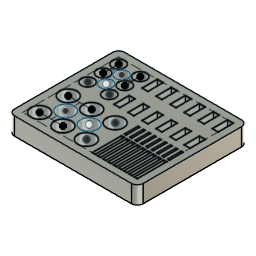
microSD-SD-flashdrive-AA-AAA holder final version. v1 (Autodesk Fusion 360 design; units mm, degrees)
Autodesk Fusion 360 part; units mm, degrees
sketch "Sketch1" plane through (0, 0, 0) normal (0, 0, 1) x (1, 0, 0)
  line L0 (55, 47) -> (-55, 47)
  line L1 (-55, 47) -> (-55, -47)
  line L2 (-55, -47) -> (55, -47)
  line L3 (55, -47) -> (55, 47)
  line L4 (55, 47) -> (-55, -47) construction
  line L5 (-55, 47) -> (55, -47) construction
  dimension "d1" = 110
  dimension "d2" = 94
  constraint horizontal L0
  constraint perpendicular L0 L1
  constraint parallel L0 L2
  constraint parallel L1 L3
  constraint coincident L4 origin
  constraint coincident L5 origin
  measures "d1" distance of L0.start L0.end
  measures "d2" distance of L0.end L1.end
extrude "Extrude1" add sketch "Sketch1" along normal blind 15
sketch "Sketch2" plane through (0, 0, 15) normal (0, 0, 1) x (-1, 0, 0)
  line L0 (-55, 47) -> (-55, -47)
  line L1 (-55, -47) -> (55, -47)
  line L2 (55, -47) -> (55, 47)
  line L3 (55, 47) -> (-55, 47)
  line L4 (49, -41) -> (-49, -41) construction
  line L5 (-49, -41) -> (-49, 41) construction
  line L6 (-49, 41) -> (49, 41) construction
  line L7 (49, 41) -> (49, -41) construction
  line L8 (-49, -41) -> (-44, -41)
  line L9 (-44, -41) -> (-44, -28)
  line L10 (-44, -28) -> (-49, -28)
  line L11 (-49, -28) -> (-49, -41)
  line L12 (-32, -41) -> (-32, -28)
  line L13 (-32, -28) -> (-37, -28)
  line L14 (-37, -28) -> (-37, -41)
  line L15 (-37, -41) -> (-32, -41)
  line L16 (-20, -41) -> (-20, -28)
  line L17 (-20, -28) -> (-25, -28)
  line L18 (-25, -28) -> (-25, -41)
  line L19 (-25, -41) -> (-20, -41)
  line L20 (-8, -41) -> (-8, -28)
  line L21 (-8, -28) -> (-13, -28)
  line L22 (-13, -28) -> (-13, -41)
  line L23 (-13, -41) -> (-8, -41)
  line L24 (4, -41) -> (4, -28)
  line L25 (4, -28) -> (-1, -28)
  line L26 (-1, -28) -> (-1, -41)
  line L27 (-1, -41) -> (4, -41)
  line L28 (16, -41) -> (16, -28)
  line L29 (16, -28) -> (11, -28)
  line L30 (11, -28) -> (11, -41)
  line L31 (11, -41) -> (16, -41)
  line L32 (-44, -17) -> (-44, -4)
  line L33 (-44, -4) -> (-49, -4)
  line L34 (-49, -4) -> (-49, -17)
  line L35 (-49, -17) -> (-44, -17)
  line L36 (-32, -17) -> (-32, -4)
  line L37 (-32, -4) -> (-37, -4)
  line L38 (-37, -4) -> (-37, -17)
  line L39 (-37, -17) -> (-32, -17)
  line L40 (-20, -17) -> (-20, -4)
  line L41 (-20, -4) -> (-25, -4)
  line L42 (-25, -4) -> (-25, -17)
  line L43 (-25, -17) -> (-20, -17)
  line L44 (-8, -17) -> (-8, -4)
  line L45 (-8, -4) -> (-13, -4)
  line L46 (-13, -4) -> (-13, -17)
  line L47 (-13, -17) -> (-8, -17)
  line L48 (4, -17) -> (4, -4)
  line L49 (4, -4) -> (-1, -4)
  line L50 (-1, -4) -> (-1, -17)
  line L51 (-1, -17) -> (4, -17)
  line L52 (16, -17) -> (16, -4)
  line L53 (16, -4) -> (11, -4)
  line L54 (11, -4) -> (11, -17)
  line L55 (11, -17) -> (16, -17)
  line L56 (-49, 2) -> (-47.5, 2)
  line L57 (-47.5, 2) -> (-47.5, 13.5)
  line L58 (-47.5, 13.5) -> (-49, 13.5)
  line L59 (-49, 13.5) -> (-49, 2)
  line L60 (-44.375, 2) -> (-42.875, 2)
  line L61 (-42.875, 2) -> (-42.875, 13.5)
  line L62 (-42.875, 13.5) -> (-44.375, 13.5)
  line L63 (-44.375, 13.5) -> (-44.375, 2)
  line L64 (-39.75, 2) -> (-38.25, 2)
  line L65 (-38.25, 2) -> (-38.25, 13.5)
  line L66 (-38.25, 13.5) -> (-39.75, 13.5)
  line L67 (-39.75, 13.5) -> (-39.75, 2)
  line L68 (-35.125, 2) -> (-33.625, 2)
  line L69 (-33.625, 2) -> (-33.625, 13.5)
  line L70 (-33.625, 13.5) -> (-35.125, 13.5)
  line L71 (-35.125, 13.5) -> (-35.125, 2)
  line L72 (-30.5, 2) -> (-29, 2)
  line L73 (-29, 2) -> (-29, 13.5)
  line L74 (-29, 13.5) -> (-30.5, 13.5)
  line L75 (-30.5, 13.5) -> (-30.5, 2)
  line L76 (-25.875, 2) -> (-24.375, 2)
  line L77 (-24.375, 2) -> (-24.375, 13.5)
  line L78 (-24.375, 13.5) -> (-25.875, 13.5)
  line L79 (-25.875, 13.5) -> (-25.875, 2)
  line L80 (-21.25, 2) -> (-19.75, 2)
  line L81 (-19.75, 2) -> (-19.75, 13.5)
  line L82 (-19.75, 13.5) -> (-21.25, 13.5)
  line L83 (-21.25, 13.5) -> (-21.25, 2)
  line L84 (-16.625, 2) -> (-15.125, 2)
  line L85 (-15.125, 2) -> (-15.125, 13.5)
  line L86 (-15.125, 13.5) -> (-16.625, 13.5)
  line L87 (-16.625, 13.5) -> (-16.625, 2)
  line L88 (-12, 2) -> (-10.5, 2)
  line L89 (-10.5, 2) -> (-10.5, 13.5)
  line L90 (-10.5, 13.5) -> (-12, 13.5)
  line L91 (-12, 13.5) -> (-12, 2)
  line L92 (-49, 16) -> (-46.5, 16)
  line L93 (-46.5, 16) -> (-46.5, 41)
  line L94 (-46.5, 41) -> (-49, 41)
  line L95 (-49, 41) -> (-49, 16)
  line L96 (-42, 16) -> (-42, 41)
  line L97 (-44.5, 16) -> (-42, 16)
  line L98 (-42, 41) -> (-44.5, 41)
  line L99 (-44.5, 41) -> (-44.5, 16)
  line L100 (-37.5, 16) -> (-37.5, 41)
  line L101 (-40, 16) -> (-37.5, 16)
  line L102 (-37.5, 41) -> (-40, 41)
  line L103 (-40, 41) -> (-40, 16)
  line L104 (-33, 16) -> (-33, 41)
  line L105 (-35.5, 16) -> (-33, 16)
  line L106 (-33, 41) -> (-35.5, 41)
  line L107 (-35.5, 41) -> (-35.5, 16)
  line L108 (-28.5, 16) -> (-28.5, 41)
  line L109 (-31, 16) -> (-28.5, 16)
  line L110 (-28.5, 41) -> (-31, 41)
  line L111 (-31, 41) -> (-31, 16)
  line L112 (-24, 16) -> (-24, 41)
  line L113 (-26.5, 16) -> (-24, 16)
  line L114 (-24, 41) -> (-26.5, 41)
  line L115 (-26.5, 41) -> (-26.5, 16)
  line L116 (-19.5, 16) -> (-19.5, 41)
  line L117 (-22, 16) -> (-19.5, 16)
  line L118 (-19.5, 41) -> (-22, 41)
  line L119 (-22, 41) -> (-22, 16)
  line L120 (-15, 16) -> (-15, 41)
  line L121 (-17.5, 16) -> (-15, 16)
  line L122 (-15, 41) -> (-17.5, 41)
  line L123 (-17.5, 41) -> (-17.5, 16)
  line L124 (-10.5, 16) -> (-10.5, 41)
  line L125 (-13, 16) -> (-10.5, 16)
  line L126 (-10.5, 41) -> (-13, 41)
  line L127 (-13, 41) -> (-13, 16)
  circle A0 centre (43.75, -35.75) radius 5.25
  circle A1 centre (25.25, -35.75) radius 5.25
  circle A2 centre (43.75, -22.5) radius 5.25
  circle A3 centre (25.25, -22.5) radius 5.25
  circle A4 centre (43.75, -9.25) radius 5.25
  circle A5 centre (25.25, -9.25) radius 5.25
  line L128 (43.75, -35.75) -> (43.75, -22.5)
  line L129 (25.25, -35.75) -> (25.25, -22.5)
  circle A6 centre (34.5, -29.125) radius 5.25
  circle A7 centre (34.5, -15.875) radius 5.25
  circle A8 centre (41.75, 33.75) radius 7.25
  circle A9 centre (21.75, 33.75) radius 7.25
  circle A10 centre (1.75, 33.75) radius 7.25
  circle A11 centre (41.75, 9.25) radius 7.25
  circle A12 centre (21.75, 9.25) radius 7.25
  circle A13 centre (1.75, 9.25) radius 7.25
  line L130 (41.75, 33.75) -> (21.75, 33.75)
  line L131 (41.75, 9.25) -> (21.75, 9.25)
  circle A14 centre (31.75, 21.5) radius 7.25
  circle A15 centre (11.75, 21.5) radius 7.25
  line L132 (31.75, 33.75) -> (31.75, 28.75)
  line L133 (31.75, 14.25) -> (31.75, 9.25)
  line L134 (43.75, -29.125) -> (39.75, -29.125)
  line L135 (29.25, -29.125) -> (25.25, -29.125)
  dimension "d5" = 98
  dimension "d6" = 82
  dimension "d7" = 6
  dimension "d8" = 6
  dimension "d9" = 5
  dimension "d10" = 13
  dimension "d13" = 12
  dimension "d14" = 24
  dimension "d15" = 1.5
  dimension "d16" = 11.5
  dimension "d17" = 6
  dimension "d20" = 4.625
  dimension "d21" = 0
  dimension "d22" = 2.5
  dimension "d23" = 25
  dimension "d24" = 2.5
  dimension "d27" = 4.5
  dimension "d28" = 0
  dimension "d29" = 10.5
  dimension "d30" = 5.25
  dimension "d31" = 5.25
  dimension "d34" = -18.5
  dimension "d35" = 13.25
  dimension "d36" = 10.5
  dimension "d39" = 0
  dimension "d40" = 13.25
  dimension "d41" = 14.5
  dimension "d42" = 7.25
  dimension "d43" = 7.25
  dimension "d46" = -20
  dimension "d47" = -24.5
  dimension "d48" = 14.5
  dimension "d51" = -20
  dimension "d52" = 0
  constraint horizontal L4
  constraint vertical L5
  constraint horizontal L6
  constraint vertical L7
  constraint horizontal L8
  constraint vertical L9
  constraint horizontal L10
  constraint vertical L11
  constraint horizontal L56
  constraint vertical L57
  constraint horizontal L58
  constraint vertical L59
  constraint coincident L5 L56.start
  constraint horizontal L92
  constraint vertical L93
  constraint horizontal L94
  constraint vertical L95
  constraint coincident L5 L92.start
  constraint coincident A0.centre L128.start
  constraint coincident A2.centre L128.end
  constraint coincident A1.centre L129.start
  constraint coincident A3.centre L129.end
  constraint midpoint L128 L134.start
  constraint midpoint L129 L135.end
  constraint coincident A8.centre L130.start
  constraint coincident A9.centre L130.end
  constraint coincident A11.centre L131.start
  constraint coincident A12.centre L131.end
  constraint midpoint L130 L132.start
  constraint midpoint L131 L133.end
  constraint coincident A14 L132.end
  constraint coincident A14 L133.start
  constraint collinear L132 L133
  constraint coincident A14.centre L132
  constraint coincident A6 L134.end
  constraint coincident A6 L135.start
  constraint collinear L134 L135
  constraint coincident A6.centre L134
  measures "d5" distance of L4.start L4.end
  measures "d6" distance of L4.start L6.end
  measures "d7" distance of L1 L4
  measures "d8" distance of L2 L7
  measures "d9" distance of L9.end L10.end
  measures "d10" distance of L8.end L9.end
  measures "d15" distance of L56.start L56.end
  measures "d16" distance of L56.end L57.end
  measures "d17" distance of L33 L56
  measures "d22" distance of L92.start L92.end
  measures "d23" distance of L92.end L93.end
  measures "d24" distance of L58 L92
  measures "d29" diameter of A0
  measures "d30" distance of L4 A0.centre
  measures "d31" distance of L7 A0.centre
  measures "d36" diameter of A6
  measures "d41" diameter of A8
  measures "d42" distance of L6 A8.centre
  measures "d43" distance of L7 A8.centre
  measures "d48" diameter of A14
extrude "Extrude2" cut sketch "Sketch2" against normal blind 10 contours L8 L9 L10 L11 | L12 L13 L14 L15 | L16 L17 L18 L19 | L20 L21 L22 L23 | L24 L25 L26 L27 | L28 L29 L30 L31 | L32 L33 L34 L35 | L36 L37 L38 L39 | L40 L41 L42 L43 | L44 L45 L46 L47 | L48 L49 L50 L51 | L52 L53 L54 L55
extrude "Extrude3" cut sketch "Sketch2" against normal blind 7 contours L56 L57 L58 L59 | L60 L61 L62 L63 | L64 L65 L66 L67 | L68 L69 L70 L71 | L72 L73 L74 L75 | L76 L77 L78 L79 | L80 L81 L82 L83 | L84 L85 L86 L87 | L88 L89 L90 L91
extrude "Extrude4" cut sketch "Sketch2" against normal blind 8 contours L92 L93 L94 L95 | L96 L97 L98 L99 | L100 L101 L102 L103 | L104 L105 L106 L107 | L108 L109 L110 L111 | L112 L113 L114 L115 | L116 L117 L118 L119 | L120 L121 L122 L123 | L124 L125 L126 L127
extrude "Extrude5" cut sketch "Sketch2" against normal blind 10 contours A0 | A1 | A2 | A3 | A4 | A5 | A6 | A7 | A8 | A9 | A10 | A11 | A12 | A13 | A14 | A15
fillet "Fillet1" radius 5 4 edges at (55, -47, 7.5) (55, 47, 7.5) (-55, 47, 7.5) (-55, -47, 7.5)
